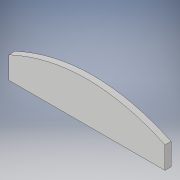
# Autodesk Inventor part: Spar-Bulkhead
Saved by Autodesk Inventor 2018 (Build 220112000, 112)
## iProperties
Created: 2018-08-08
Part Number: Spar-Bulkhead
Material: Generic
Document SubType Name: Modeling
Designer: Michael Gunderman
Density: 1 g/cm^3
Appearance: Default
Author: Michael Gunderman
Autodesk Inventor part; units mm, degrees
ref_plane "YZ Plane" through (0, 0, 0) normal (1, 0, 0) x (0, 1, 0)
ref_plane "XZ Plane" through (0, 0, 0) normal (0, 1, 0) x (-1, 0, 0)
ref_plane "XY Plane" through (0, 0, 0) normal (0, 0, 1) x (1, 0, 0)
sketch "Sketch2" plane through (0, 0, 0) normal (0, 0, 1) x (1, 0, 0)
  line L0 (0, 0) -> (-127, 0)
  line L1 (-127, 0) -> (-127, 35.9784)
  line L2 (0, 0) -> (127, 0)
  line L3 (127, 0) -> (127, 35.9784)
  spline S0 degree 2 poles (-127, 35.9784) (0, 94.576) (127, 35.9784) knots 0 0 0 1 1 1
  point P0 (0, 65.2772)
  dimension "d5" = 127
  dimension "d6" = 127
  constraints: 8 end point, 2 perpendicular, 1 point on line, 3 other
  measures "d5" distance of L0.start L0.end
  measures "d6" distance of L0.start L2.end
extrude "Extrusion1" add sketch "Sketch2" along normal blind 10
body "Solid1"
